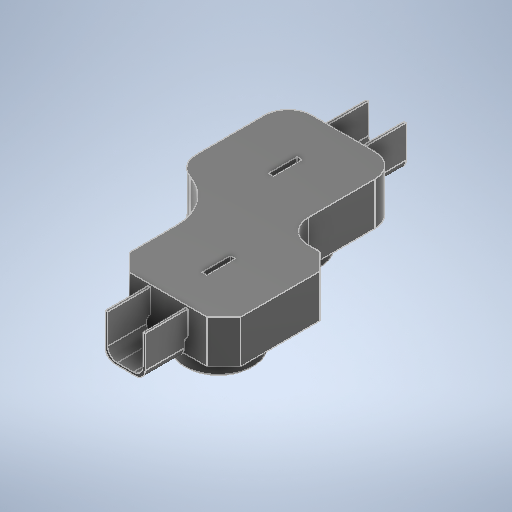
# Autodesk Inventor part: Kailh Choc Hotswap Socket Negative
Saved by Autodesk Inventor 2025 (Build 290162000, 162)
## iProperties
Created: 2025-11-22
Part Number: Kailh Choc Hotswap Socket Negative
Material: Generic
Document SubType Name: Modeling
Designer: User
Density: 1 g/cm^3
Appearance: Smooth - Black
Author: User
Autodesk Inventor part; units mm, degrees
ref_plane "YZ Plane" through (0, 0, 0) normal (1, 0, 0) x (0, 1, 0)
ref_plane "XZ Plane" through (0, 0, 0) normal (0, 1, 0) x (-1, 0, 0)
ref_plane "XY Plane" through (0, 0, 0) normal (0, 0, 1) x (1, 0, 0)
sketch "Sketch1" plane through (0, 0, 0) normal (0, 1, 0) x (-1, 0, 0)
  line L0 (0, 0) -> (-3.8165, 0)
  line L1 (-3.8165, 0) -> (-3.1049, -0.7116)
  line L2 (-3.1049, -0.7116) -> (-3.1049, -2.701)
  arc A0 (-3.1049, -2.701) -> (-1.6284, -4.75) centre (-0.9449, -2.701) ccw
  line L3 (-0.9449, -5.6986) -> (-0.9449, -8.55)
  line L4 (-1.9449, -9.55) -> (-4.5949, -9.55)
  line L5 (-5.5949, -8.55) -> (-5.5949, -5.75)
  line L6 (-6.5949, -4.75) -> (-7.0833, -4.75)
  line L7 (-7.0833, -4.75) -> (-7.7949, -4.0384)
  line L8 (-7.7949, -4.0384) -> (-7.7949, -0.7116)
  line L9 (-7.7949, -0.7116) -> (-7.0833, 0)
  line L10 (-7.0833, 0) -> (-3.8165, 0)
  circle A1 centre (-5.4499, -2.1243) radius 1.45
  circle A2 centre (-3.2499, -7.1243) radius 1.45
  arc A3 (-0.9449, -5.6986) -> (-1.6284, -4.75) centre (-1.9449, -5.6986) ccw
  arc A4 (-5.5949, -5.75) -> (-6.5949, -4.75) centre (-6.5949, -5.75) ccw
  arc A5 (-1.9449, -9.55) -> (-0.9449, -8.55) centre (-1.9449, -8.55) ccw
  arc A6 (-5.5949, -8.55) -> (-4.5949, -9.55) centre (-4.5949, -8.55) ccw
  point P0 (-0.9449, -4.861)
  point P1 (-5.5949, -7.15)
  point P2 (-5.4499, 0)
  point P3 (-6.8391, -4.75)
  point P4 (-0.9449, -7.1243)
  dimension "d0" = 5
  dimension "d1" = 2.2
  dimension "d2" = 2.9
  dimension "d3" = 4.75
  dimension "d4" = 4.65
  dimension "d6" = 4.69
  dimension "d8" = 6.85
  dimension "d9" = 9.55
  dimension "d10" = 135
  dimension "d11" = 135
  dimension "d12" = 135
  dimension "d13" = 1
  dimension "d14" = 1
  constraints: 22 end point, 11 point on circle, 9 tangent, 7 centre point, 6 perpendicular, 4 midpoint, 3 equal radius, 2 horizontal alignment, 2 vertical, 1 horizontal, 1 line through centre, 1 parallel, 1 point on line, 1 vertical alignment
  measures "d0" vertical distance of A2.centre A1.centre
  measures "d1" horizontal distance of A2.centre A1.centre
  measures "d2" diameter of A1
  measures "d3" distance between parallel lines of L6 L10
  measures "d4" distance from line of L3 point (-5.595, -7.15)
  measures "d6" distance between parallel lines of L8 L2
  measures "d8" distance between parallel lines of L3 L8
  measures "d9" distance between parallel lines of L10 L4
  measures "d10" angle of L6 L7
  measures "d11" angle of L8 L9
  measures "d12" angle of L1 L10
  measures "d13" radius of A3
  measures "d14" radius of A5
extrude "Extrusion1" add sketch "Sketch1" along normal blind 1.8 contours L1 L2 A0 A3 L3 A5 L4 A6 L5 A4 L6 L7 L8 L9 L10 | A1 | A2
extrude "Extrusion2" add sketch "Sketch1" against normal blind 1.25 contours A1 | A2
chamfer "Chamfer1" distance 0.1 angle 45 2 edges at (6.8999, -1.25, -2.1243) (4.6999, -1.25, -7.1243)
sketch "Sketch2" plane through (3.8165, 0, 0) normal (0, 0, 1) x (1, 0, 0)
  line L0 (1.7784, 1.8) -> (2.7784, 1.8) projected
  line L1 (2.4734, -0.05) -> (0.7934, -0.05)
  line L2 (0.7784, 0) -> (0.7784, 1.8) projected
  line L3 (3.2668, 0) -> (3.2668, 1.8) projected
  line L4 (0, 0) -> (0, 1.8) projected
  line L5 (0, 1.8) -> (3.2668, 1.8) projected
  line L6 (2.4734, -0.05) -> (2.4734, 1.7)
  line L7 (0.7934, -0.05) -> (0.7934, 1.7)
  line L8 (0.8934, 1.7) -> (0.8934, 0.05)
  line L9 (0.8934, 0.05) -> (2.3734, 0.05)
  line L10 (2.3734, 0.05) -> (2.3734, 1.7)
  line L11 (2.4734, 1.7) -> (2.3734, 1.7)
  line L12 (0.8934, 1.7) -> (0.7934, 1.7)
  point P0 (-3.8165, 0)
  dimension "d24" = 1.68
  dimension "d26" = 1.85
  dimension "d27" = 0.1
  dimension "d28" = 0.7934
  dimension "d29" = 0.7934
  dimension "d30" = 0.1
  dimension "d31" = 0.1
  constraints: 16 end point, 2 vertical, 1 collinear, 1 horizontal, 1 parallel, 1 perpendicular, 1 other
  measures "d24" distance of L1.start L1.end
  measures "d26" distance between parallel lines of L5 L1
  measures "d27" distance from line of L6.end L0
  measures "d28" distance between parallel lines of L6 L3
  measures "d29" distance between parallel lines of L4 L7
  measures "d30" distance between parallel lines of L1 L9
  measures "d31" distance between parallel lines of L10 L6
extrude "Extrusion3" add sketch "Sketch2" along normal blind 1.8
sketch "Sketch3" plane through (4.6099, 0, 0) normal (-1, 0, 0) x (0, 0, 1)
  line L0 (0, -0.05) -> (1.8, -0.05) projected
  line L1 (0.16, -0.05) -> (0.16, 0.54)
  line L2 (0, 0) -> (0, 1.7) projected
  arc A0 (0.16, 0.54) -> (0, 0.7) centre (0, 0.54) ccw
  line L3 (0, 0) -> (0, 1.8) projected
  line L4 (0, 0) -> (0, 1.7) projected
  line L5 (0, 0) -> (0, -0.05) projected
  line L6 (0, -0.05) -> (1.8, -0.05) projected
  line L7 (1.8, 1.7) -> (1.8, -0.05) projected
  line L8 (0, 1.7) -> (1.8, 1.7) projected
  point P0 (0, 0)
  dimension "d34" = 0.16
  dimension "d54" = 0.75
  constraints: 2 end point, 2 point on circle, 2 point on line, 1 centre point, 1 line through centre, 1 tangent, 1 vertical
  measures "d34" distance between parallel lines of L2 L1
extrude "Extrusion4" cut sketch "Sketch3" against normal through all contours L5 L2 A0 L1 L0
sketch "Sketch4" plane through (4.5949, 0, -9.55) normal (0, 0, -1) x (-1, 0, 0)
  line L0 (2.165, -0.05) -> (0.485, -0.05)
  line L1 (2.165, -0.05) -> (2.165, 1.7)
  line L2 (0.485, -0.05) -> (0.485, 1.7)
  line L3 (0.585, 1.7) -> (0.585, 0.05)
  line L4 (0.585, 0.05) -> (2.065, 0.05)
  line L5 (2.065, 0.05) -> (2.065, 1.7)
  line L6 (2.165, 1.7) -> (2.065, 1.7)
  line L7 (0.585, 1.7) -> (0.485, 1.7)
  line L8 (2.65, 0) -> (2.65, 1.8) projected
  line L9 (0, 1.8) -> (2.65, 1.8) projected
  line L10 (0, 0) -> (0, 1.8) projected
  point P0 (4.5949, 0)
  dimension "d37" = 1.68
  dimension "d42" = 0.1
  dimension "d43" = 0.1
  dimension "d44" = 0.485
  dimension "d45" = 0.485
  dimension "d46" = 1.85
  dimension "d47" = 0.1
  constraints: 16 end point, 2 horizontal, 2 vertical, 1 collinear, 1 parallel, 1 other
  measures "d37" distance of L0.start L0.end
  measures "d42" distance between parallel lines of L0 L4
  measures "d43" distance between parallel lines of L5 L1
  measures "d44" distance between parallel lines of L8 L1
  measures "d45" distance between parallel lines of L2 L10
  measures "d46" distance between parallel lines of L9 L0
  measures "d47" distance between parallel lines of L9 L6
extrude "Extrusion5" add sketch "Sketch4" along normal blind 1.8
sketch "Sketch5" plane through (2.4299, 0, -9.55) normal (-1, 0, 0) x (0, 0, 1)
  line L0 (0, -0.05) -> (0, 0) projected
  line L1 (0, 1.7) -> (0, 0) projected
  line L2 (0, 1.7) -> (-1.8, 1.7) projected
  line L3 (-1.8, -0.05) -> (-1.8, 1.7) projected
  line L4 (0, -0.05) -> (-1.8, -0.05) projected
  line L5 (-0.16, -0.05) -> (-0.16, 0.54)
  arc A0 (0, 0.7) -> (-0.16, 0.54) centre (0, 0.54) ccw
  point P0 (9.55, 0)
  point P1 (-1.867, -0.613)
  point P2 (-1.867, -0.6608)
  point P3 (0, -0.025)
  dimension "d51" = 0.16
  dimension "d55" = 0.75
  constraints: 2 end point, 2 point on circle, 2 point on line, 1 centre point, 1 line through centre, 1 midpoint, 1 tangent, 1 vertical
  measures "d51" distance from line of point (0, -0.025) L5
extrude "Extrusion6" cut sketch "Sketch5" against normal through all contours L4 L5 A0 L1 L0
sketch "Sketch6" plane through (5.4499, -1.25, -2.1243) normal (0, -1, 0) x (1, 0, 0)
  line L0 (0.1, 0.6) -> (-0.1, 0.6)
  line L1 (-0.1, 0.6) -> (-0.1, -0.6)
  line L2 (-0.1, -0.6) -> (0.1, -0.6)
  line L3 (0.1, -0.6) -> (0.1, 0.6)
  line L4 (-2.1, -4.4) -> (-2.3, -4.4)
  line L5 (-2.3, -4.4) -> (-2.3, -5.6)
  line L6 (-2.3, -5.6) -> (-2.1, -5.6)
  line L7 (-2.1, -5.6) -> (-2.1, -4.4)
  circle A0 centre (0, 0) radius 1.35 projected
  circle A1 centre (-2.2, -5) radius 1.35 projected
  point P0 (-5.4499, 2.1243)
  point P1 (0.1, 0)
  point P2 (0, 0.6)
  point P3 (-2.1, -5)
  point P4 (-2.2, -4.4)
  dimension "d56" = 1.2
  dimension "d57" = 0.2
  dimension "d58" = 1.2
  dimension "d59" = 0.2
  constraints: 16 end point, 4 midpoint, 4 parallel, 2 horizontal, 2 horizontal alignment, 2 perpendicular, 2 vertical alignment
  measures "d56" distance of L2.end L0.start
  measures "d57" distance of L0.start L0.end
  measures "d58" distance of L6.end L4.start
  measures "d59" distance of L4.start L4.end
extrude "Extrusion7" cut sketch "Sketch6" against normal through all contours L3 L2 L1 L0 | L7 L6 L5 L4
chamfer "Chamfer2" distance 0.2 angle 45 8 edges at (5.5499, -1.25, -2.1243) (5.4499, -1.25, -1.5243) (5.3499, -1.25, -2.1243) (5.4499, -1.25, -2.7243) (3.3499, -1.25, -7.1243) (3.2499, -1.25, -6.5243) (3.1499, -1.25, -7.1243) (3.2499, -1.25, -7.7243)
fillet "Fillet1" radius 0.4 8 edges at (4.6099, -0.05, 0.98) (6.2899, -0.05, 0.98) (6.1899, 0.05, 0.98) (4.7099, 0.05, 0.98) (2.4299, -0.05, -10.53) (4.1099, -0.05, -10.53) (4.0099, 0.05, -10.53) (2.5299, 0.05, -10.53)
equation "\"d11\" = d10"
equation "\"d29\" = d28"
body "Solid1"
